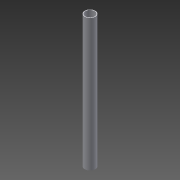
# Autodesk Inventor part: Rura_oparcia
Saved by Autodesk Inventor 2014 SP2 (Build 180246200, 246)
## iProperties
Created: 2015-11-22
Part Number: Rura_oparcia
Material: Aluminium AW-7020
Document SubType Name: Modelowanie
Designer: graaapsik
Density: 2.78 g/cm^3
Appearance: Aluminium AW-7020
Author: graaapsik
Autodesk Inventor part; units mm, degrees
ref_plane "YZ Plane" through (0, 0, 0) normal (1, 0, 0) x (0, 1, 0)
ref_plane "XZ Plane" through (0, 0, 0) normal (0, 1, 0) x (-1, 0, 0)
ref_plane "XY Plane" through (0, 0, 0) normal (0, 0, 1) x (1, 0, 0)
sketch "Szkic2" plane through (0, 0, 0) normal (0, 0, 1) x (1, 0, 0)
  circle A0 centre (0, 0) radius 16
  dimension "d4" = 32
  constraints: 1 centre point, 1 coincident
  measures "d4" diameter of A0
extrude "Wyciągnięcie proste2" add sketch "Szkic2" along normal blind 400
shell "Skorupa2" thickness 2 removed faces 2 at (4.7224, 2.4785, 400) at (4.7224, 2.4785, 0)
sketch "Szkic3" plane through (0, 0, 0) normal (0, 1, 0) x (-1, 0, 0)
  line L0 (-16, 0) -> (16, 0) construction
  line L1 (0, 0) -> (0, 395.7207) construction
  point P0 (0, 50)
  point P1 (0, 170)
  point P2 (0, 260)
  point P3 (0, 350)
  dimension "d8" = 90
  dimension "d9" = 90
  dimension "d10" = 120
  dimension "d11" = 50
  constraints: 4 point on line, 2 end point, 1 perpendicular
  measures "d8" distance of point (0, 260) point (0, 350)
  measures "d9" distance of point (0, 170) point (0, 260)
  measures "d10" distance of point (0, 50) point (0, 170)
  measures "d11" distance from line of L0 point (0, 50)
hole "Otwór1" at (0, 0, 50) at (0, 0, 170) at (0, 0, 260) at (0, 0, 350) direction (0, 1, 0) diameter 6 depth 16 tip angle 118
equation "\"PromieńGięcia\" = Grubość"
equation "\"SzerokośćGięciaPodcięcia\" = Grubość"
equation "\"GłębokośćGięciaPodcięcia\" = 0.5 * Grubość"
equation "\"RozmiarPodcięciaNarożnika\" = 4 * Grubość"
equation "\"MinimalnaPozostałość\" = 2 * Grubość"
equation "\"PromieńPrzejścia\" = PromieńGięcia"
equation "\"Rozmiar_promienia_Jacobiego\" = PromieńGięcia"
equation "\"Wielk_odstępu\" = Grubość"
equation "\"Grubość\" = 0.5"
